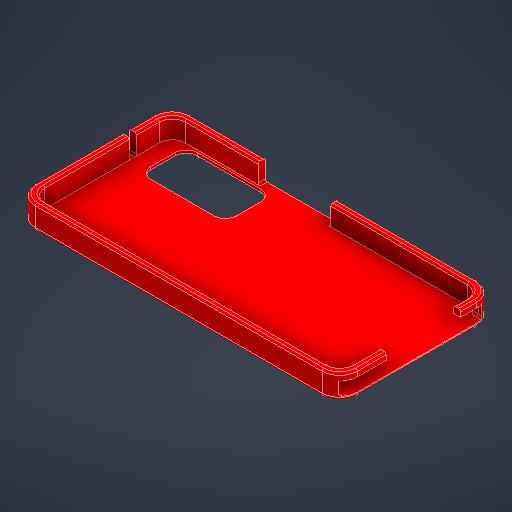
# Autodesk Inventor part: CarcasaBase
Saved by Autodesk Inventor 2026 (Build 300175000, 175)
## iProperties
Created: 2025-06-24
Part Number: CarcasaBase
Material: Genérico
Document SubType Name: Modeling
Designer: Estudiante
Density: 1 g/cm^3
Appearance: Valor por defecto
Author: Estudiante
Autodesk Inventor part; units mm, degrees
ref_plane "YZ Plane" through (0, 0, 0) normal (1, 0, 0) x (0, 1, 0)
ref_plane "XZ Plane" through (0, 0, 0) normal (0, 1, 0) x (-1, 0, 0)
ref_plane "XY Plane" through (0, 0, 0) normal (0, 0, 1) x (1, 0, 0)
sketch "Boceto1" plane through (0, 0, 0) normal (0, 1, 0) x (-1, 0, 0)
  line L0 (0, 0) -> (173, 0)
  line L1 (173, 0) -> (173, -83)
  line L2 (173, -83) -> (0, -83)
  line L3 (0, -83) -> (0, 0)
  dimension "d0" = 173
  dimension "d1" = 83
  constraints: 8 end point, 2 parallel, 1 horizontal, 1 perpendicular
  measures "d0" distance of L1.end L2.end
  measures "d1" distance of L0.end L1.end
extrude "Extrusión1" add sketch "Boceto1" along normal blind 13.2
fillet "Empalme1" radius 9.5 4 edges at (-173, 6.6, -83) (0, 6.6, -83) (-173, 6.6, 0) (0, 6.6, 0)
sketch "Boceto2" plane through (0, 13.2, 0) normal (0, 1, 0) x (1, 0, 0)
  line L0 (0, 0) -> (0, 3.75)
  line L1 (0, 9.5) -> (0, 73.5) projected
  line L2 (0, 3.75) -> (-3.75, 3.75)
  line L3 (-3.75, 3.75) -> (-169.25, 3.75)
  line L4 (-169.25, 3.75) -> (-169.25, 79.25)
  line L5 (-169.25, 79.25) -> (-3.75, 79.25)
  line L6 (-3.75, 79.25) -> (-3.75, 3.75)
  line L7 (-169.25, 3.75) -> (-169.25, 10.75)
  line L8 (-169.25, 10.75) -> (-162.25, 10.75)
  circle A0 centre (-162.25, 10.75) radius 7
  line L9 (-169.25, 79.25) -> (-162.25, 79.25)
  line L10 (-162.25, 79.25) -> (-162.25, 72.25)
  circle A1 centre (-162.25, 72.25) radius 7
  line L11 (-3.75, 3.75) -> (-3.75, 10.75)
  line L12 (-3.75, 10.75) -> (-10.75, 10.75)
  circle A2 centre (-10.75, 10.75) radius 7
  line L13 (-3.75, 79.25) -> (-10.75, 79.25)
  line L14 (-10.75, 79.25) -> (-10.75, 72.25)
  circle A3 centre (-10.75, 72.25) radius 7
  point P0 (-169.25, 72.25)
  point P1 (-162.25, 3.75)
  point P2 (-10.75, 3.75)
  point P3 (-3.75, 72.25)
  dimension "d5" = 3.75
  dimension "d6" = 3.75
  dimension "d7" = 165.5
  dimension "d8" = 75.5
  dimension "d9" = 7
  dimension "d10" = 7
  dimension "d11" = 7
  dimension "d12" = 7
  dimension "d13" = 7
  dimension "d14" = 7
  dimension "d15" = 7
  dimension "d16" = 7
  constraints: 28 end point, 6 perpendicular, 4 coincident, 4 point on line, 2 parallel, 1 collinear, 1 horizontal, 12 other
  measures "d5" distance of L0.start L0.end
  measures "d6" distance of L0.end L2.end
  measures "d7" distance of L4.end L5.end
  measures "d8" distance of L3.end L4.end
  measures "d9" distance of L3.end L7.end
  measures "d10" distance of L7.end L8.end
  measures "d11" distance of L4.end L9.end
  measures "d12" distance of L9.end L10.end
  measures "d13" distance of L2.end L11.end
  measures "d14" distance of L11.end L12.end
  measures "d15" distance of L5.end L13.end
  measures "d16" distance of L13.end L14.end
extrude "Extrusión2" cut sketch "Boceto2" against normal blind 10.7 contours L3 A0 L4 A1 L5 A3 L6 A2 | A2 | A0 | A3 | A1
sketch "Boceto3" plane through (0, 0, 0) normal (0, -1, 0) x (1, 0, 0)
  line L0 (0, 0) -> (0, -65.5)
  line L1 (0, -9.5) -> (0, -73.5) projected
  line L2 (0, -65.5) -> (-137.5, -65.5)
  line L3 (-137.5, -65.5) -> (-137.5, -53)
  line L4 (-137.5, -53) -> (-114.5, -53)
  line L5 (-114.5, -53) -> (-160.5, -53)
  line L6 (-160.5, -53) -> (-160.5, -78)
  line L7 (-160.5, -78) -> (-114.5, -78)
  line L8 (-114.5, -78) -> (-114.5, -53)
  line L9 (-114.5, -78) -> (-114.5, -72)
  line L10 (-114.5, -72) -> (-120.5, -72)
  circle A0 centre (-120.5, -72) radius 6
  line L11 (-114.5, -53) -> (-114.5, -59)
  line L12 (-114.5, -59) -> (-120.5, -59)
  circle A1 centre (-120.5, -59) radius 6
  line L13 (-160.5, -78) -> (-160.5, -72)
  line L14 (-160.5, -72) -> (-154.5, -72)
  circle A2 centre (-154.5, -72) radius 6
  line L15 (-160.5, -53) -> (-154.5, -53)
  line L16 (-154.5, -53) -> (-154.5, -59)
  circle A3 centre (-154.5, -59) radius 6
  point P0 (-160.5, -59)
  point P1 (-154.5, -78)
  point P2 (-120.5, -78)
  point P3 (-120.5, -53)
  dimension "d19" = 65.5
  dimension "d20" = 137.5
  dimension "d21" = 12.5
  dimension "d22" = 23
  dimension "d23" = 46
  dimension "d24" = 25
  dimension "d25" = 6
  dimension "d26" = 6
  dimension "d27" = 6
  dimension "d28" = 6
  dimension "d29" = 6
  dimension "d30" = 6
  dimension "d31" = 6
  dimension "d32" = 6
  constraints: 32 end point, 8 perpendicular, 5 point on line, 4 coincident, 2 parallel, 1 horizontal, 12 other
  measures "d19" distance of L0.start L0.end
  measures "d20" distance of L0.end L2.end
  measures "d21" distance of L2.end L3.end
  measures "d22" distance of L3.end L4.end
  measures "d23" distance of L7.end L6.end
  measures "d24" distance of L6.end L5.end
  measures "d25" distance of L7.end L9.end
  measures "d26" distance of L9.end L10.end
  measures "d27" distance of L4.end L11.end
  measures "d28" distance of L11.end L12.end
  measures "d29" distance of L6.end L13.end
  measures "d30" distance of L13.end L14.end
  measures "d31" distance of L5.end L15.end
  measures "d32" distance of L15.end L16.end
extrude "Extrusión3" cut sketch "Boceto3" against normal blind 2.5 contours L8 A0 L7 A2 L6 A3 L5 L3 L2 | L2 L3 L4 A1 L8 | A0 | A1 | A3 | A2
sketch "Boceto5" plane through (0, 0, -9.5) normal (1, 0, 0) x (0, 0, -1)
  line L0 (-9.5, 0) -> (15.5, 0)
  line L1 (0, 0) -> (64, 0) projected
  line L2 (15.5, 0) -> (15.5, 2.5)
  line L3 (64, 13.2) -> (0, 13.2) projected
  line L4 (15.5, 2.5) -> (55.5, 2.5)
  line L5 (15.5, 2.5) -> (15.5, 13.2)
  line L6 (55.5, 2.5) -> (55.5, 13.2)
  dimension "d38" = 25
  dimension "d39" = 2.5
  dimension "d41" = 40
  constraints: 10 end point, 3 perpendicular, 3 point on line, 1 horizontal
  measures "d38" distance of L0.start L0.end
  measures "d39" distance of L0.end L2.end
  measures "d41" distance of L2.end L4.end
extrude "Extrusión4" cut sketch "Boceto5" against normal blind 13.2
sketch "Boceto6" plane through (-173, 0, -73.5) normal (-1, 0, 0) x (0, 0, 1)
  line L0 (73.5, 0) -> (17.5, 0)
  line L1 (0, 0) -> (64, 0) projected
  line L2 (17.5, 0) -> (17.5, 2.5)
  line L3 (17.5, 2.5) -> (13.5, 2.5)
  line L4 (13.5, 2.5) -> (13.5, 13.2)
  line L5 (0, 13.2) -> (64, 13.2) projected
  line L6 (17.5, 2.5) -> (17.5, 13.2)
  point P0 (29.3, 13.9)
  dimension "d44" = 56
  dimension "d45" = 2.5
  dimension "d46" = 4
  constraints: 10 end point, 3 point on line, 3 vertical, 1 perpendicular
  measures "d44" distance of L0.start L0.end
  measures "d45" distance of L0.end L2.end
  measures "d46" distance of L2.end L3.end
extrude "Extrusión5" cut sketch "Boceto6" against normal blind 10.7
sketch "Boceto7" plane through (-9.5, 0, -83) normal (0, 0, -1) x (-1, 0, 0)
  line L0 (-9.5, 13.2) -> (-9.5, 0) projected
  line L1 (-9.5, 0) -> (74.5, 0)
  line L2 (0, 0) -> (154, 0) projected
  line L3 (74.5, 0) -> (74.5, 2.5)
  line L4 (0, 13.2) -> (154, 13.2) projected
  line L5 (74.5, 2.5) -> (74.5, 13.2)
  line L6 (74.5, 2.5) -> (113.5, 2.5)
  line L7 (1.25, 2.5) -> (152.75, 2.5) projected
  line L8 (113.5, 2.5) -> (113.5, 13.2)
  line L9 (113.5, 13.2) -> (74.5, 13.2)
  dimension "d132" = 84
  dimension "d133" = 2.5
  dimension "d134" = 10.7
  dimension "d135" = 39
  dimension "d136" = 10.7
  constraints: 12 end point, 4 point on line, 1 perpendicular
  measures "d132" distance of L0.end L1.end
  measures "d133" distance of L1.end L3.end
  measures "d134" distance of L3.end L5.end
  measures "d135" distance of L3.end L6.end
  measures "d136" distance of L6.end L8.end
sketch "Boceto12" plane through (0, 2.5, 0) normal (0, 1, 0) x (1, 0, 0)
  line L0 (6.4, 0) -> (6.4, 2.5)
  line L1 (-0.1, 8.5) -> (-0.1, 76.5)
  line L2 (6.4, 2.5) -> (3.9, 2.5)
  line L3 (3.9, 2.5) -> (-164.1, 2.5)
  line L4 (-164.1, 2.5) -> (-164.1, 77.5)
  line L5 (-164.1, 77.5) -> (3.9, 77.5)
  line L6 (3.9, 77.5) -> (3.9, 2.5)
  line L7 (-164.1, 2.5) -> (-164.1, 9.5)
  line L8 (-164.1, 9.5) -> (-157.1, 9.5)
  circle A0 centre (-157.1, 9.5) radius 7
  line L9 (-164.1, 77.5) -> (-157.1, 77.5)
  line L10 (-157.1, 77.5) -> (-157.1, 70.5)
  circle A1 centre (-157.1, 70.5) radius 7
  line L11 (3.9, 2.5) -> (3.9, 9.5)
  line L12 (3.9, 9.5) -> (-3.1, 9.5)
  circle A2 centre (-3.1, 9.5) radius 7
  line L13 (3.9, 77.5) -> (-3.1, 77.5)
  line L14 (-3.1, 77.5) -> (-3.1, 70.5)
  circle A3 centre (-3.1, 70.5) radius 7
  point P0 (0, 0)
  point P1 (-157.1, 2.5)
  point P2 (-3.1, 2.5)
  point P3 (-0.1, 64.1754)
  point P4 (-164.1, 70.5)
  point P5 (-0.1, 15.8246)
  point P6 (-0.1, 76.5)
  point P7 (3.9, 70.5)
  dimension "d90" = 2.5
  dimension "d91" = 2.5
  dimension "d92" = 168
  dimension "d93" = 75
  dimension "d94" = 7
  dimension "d95" = 7
  dimension "d96" = 7
  dimension "d97" = 7
  dimension "d98" = 7
  dimension "d99" = 7
  dimension "d100" = 7
  dimension "d101" = 7
  constraints: 30 end point, 6 perpendicular, 4 coincident, 4 point on line, 3 parallel, 1 horizontal, 12 other
  measures "d90" distance of L0.start L0.end
  measures "d91" distance of L0.end L11.start
  measures "d92" distance of L5.start L6.start
  measures "d93" distance of L3.end L5.start
  measures "d94" distance of L3.end L8.start
  measures "d95" distance of L8.start L8.end
  measures "d96" distance of L5.start L10.start
  measures "d97" distance of L10.start L10.end
  measures "d98" distance of L11.start L11.end
  measures "d99" distance of L11.end L12.end
  measures "d100" distance of L6.start L14.start
  measures "d101" distance of L14.start L14.end
extrude "Extrusión10" cut sketch "Boceto12" along normal blind 7 contours L12 A2 L1 | L1 A2 L12 | A2 L3 A0 L4 A1 L5 A3 L1 | L1 A3 L6 A2 | A3 | A0 | A1
sketch "Boceto9" plane through (-163.5, 0, 0) normal (0, 0, 1) x (1, 0, 0)
  line L0 (154, 0) -> (0, 0) projected
  line L1 (152.75, 2.5) -> (1.25, 2.5) projected
  line L2 (163.5, 0) -> (243.5, 0)
  line L3 (243.5, 0) -> (243.5, 0)
  line L4 (243.5, 0) -> (243.5, 2.5)
  line L5 (243.5, 0) -> (243.5, 2.5)
  line L6 (243.5, 2.5) -> (243.5, 2.5)
  line L7 (243.5, 2.5) -> (243.5, 13.2)
  line L8 (243.5, 13.2) -> (243.5, 13.2)
  line L9 (243.5, 13.2) -> (243.5, 2.5)
  point P0 (243, 2.5)
  point P1 (191, 2.5)
  dimension "d117" = 80
  dimension "d118" = 0
  dimension "d119" = 10.7
  constraints: 16 end point, 6 point on line, 5 perpendicular, 1 collinear
  measures "d117" distance of L2.start L2.end
  measures "d118" distance of L2.end L3.end
  measures "d119" distance of L4.end L7.end
sketch "Boceto10" plane through (0, 0, 0) normal (0, -1, 0) x (1, 0, 0)
  line L0 (0, 0) -> (-102.5, 0)
  line L1 (-163.5, 0) -> (-9.5, 0) projected
  line L2 (-102.5, 0) -> (-102.5, -40)
  line L3 (-102.5, -40) -> (-102.5, -39.99)
  line L4 (-102.5, -39.99) -> (-102.51, -39.99)
  line L5 (-102.51, -39.99) -> (-102.49, -39.99)
  line L6 (-102.49, -39.99) -> (-102.49, -40.01)
  line L7 (-102.49, -40.01) -> (-102.51, -40.01)
  line L8 (-102.51, -40.01) -> (-102.51, -39.99)
  line L9 (-102.51, -40.01) -> (-102.5, -40.01)
  line L10 (-102.5, -40.01) -> (-102.5, -40)
  circle A0 centre (-102.5, -40) radius 0.01
  line L11 (-102.51, -39.99) -> (-102.51, -40)
  line L12 (-102.51, -40) -> (-102.5, -40)
  circle A1 centre (-102.5, -40) radius 0.01
  line L13 (-102.49, -40.01) -> (-102.49, -40)
  line L14 (-102.49, -40) -> (-102.5, -40)
  circle A2 centre (-102.5, -40) radius 0.01
  line L15 (-102.49, -39.99) -> (-102.49, -40)
  line L16 (-102.49, -40) -> (-102.5, -40)
  circle A3 centre (-102.5, -40) radius 0.01
  point P0 (-102.5, -39.99)
  point P1 (-102.5, -39.99)
  point P2 (-102.5, -40.01)
  dimension "d69" = 102.5
  dimension "d70" = 40
  dimension "d71" = 0.01
  dimension "d72" = 0.01
  dimension "d73" = 0.02
  dimension "d74" = 0.02
  dimension "d75" = 0.01
  dimension "d76" = 0.01
  dimension "d77" = 0.01
  dimension "d78" = 0.01
  dimension "d79" = 0.01
  dimension "d80" = 0.01
  dimension "d81" = 0.01
  dimension "d82" = 0.01
  constraints: 32 end point, 6 perpendicular, 4 coincident, 4 midpoint, 2 parallel, 2 point on line, 1 horizontal, 1 vertical, 12 other
  measures "d69" distance of L0.start L0.end
  measures "d70" distance of L0.end L2.end
  measures "d71" distance of L2.end L3.end
  measures "d72" distance of L3.end L4.end
  measures "d73" distance of L6.end L7.end
  measures "d74" distance of L5.end L6.end
  measures "d75" distance of L7.end L9.end
  measures "d76" distance of L9.end L10.end
  measures "d77" distance of L4.end L11.end
  measures "d78" distance of L11.end L12.end
  measures "d79" distance of L6.end L13.end
  measures "d80" distance of L13.end L14.end
  measures "d81" distance of L5.end L15.end
  measures "d82" distance of L15.end L16.end
extrude "Extrusión9" cut sketch "Boceto10" against normal blind 10.7 contours A0 L14 L2 | L2 L12 A0 | L14 A0 L10 | L10 A0 L12
extrude "Extrusión11" [suppressed]
fillet "Empalme15" radius 2 8 edges at (-86.5, 0, 0) (-2.7825, 0, -2.7825) (0, 0, -41.5) (-2.7825, 0, -80.2175) (-86.5, 0, -83) (-170.2175, 0, -80.2175) (-173, 0, -41.5) (-170.2175, 0, -2.7825)
fillet "Empalme16" radius 1 8 edges at (-116.2574, 0, -54.7574) (-114.5, 0, -65.5) (-116.2574, 0, -76.2426) (-137.5, 0, -78) (-158.7426, 0, -76.2426) (-160.5, 0, -65.5) (-158.7426, 0, -54.7574) (-137.5, 0, -53)
fillet "Empalme18" radius 0.01 4 edges at (-102.4929, 0, -40.0071) (-102.5071, 0, -40.0071) (-102.5071, 0, -39.9929) (-102.4929, 0, -39.9929)
fillet "Empalme19" radius 1 10 edges at (-170.2175, 13.2, -2.7825) (-173, 13.2, -32.75) (-86.5, 13.2, 0) (-2.7825, 13.2, -2.7825) (0, 13.2, -17.25) (-2.7825, 13.2, -80.2175) (0, 13.2, -69.25) (-86.5, 13.2, -83) (-170.2175, 13.2, -80.2175) (-173, 13.2, -66.75)
fillet "Empalme20" radius 1 10 edges at (-167.1997, 13.2, -5.8003) (-169.25, 13.2, -33.375) (-86.5, 13.2, -3.75) (-5.8003, 13.2, -5.8003) (-3.75, 13.2, -17.875) (-167.1997, 13.2, -77.1997) (-169.25, 13.2, -66.125) (-86.5, 13.2, -79.25) (-5.8003, 13.2, -77.1997) (-3.75, 13.2, -68.625)
fillet "Empalme21" radius 1 5 edges at (-4.61, 2.5, -77.5) (-1.8805, 2.5, -77.393) (-159.1917, 2.5, -2.8198) (-80.1, 2.5, -2.5) (-3.0887, 2.5, -2.5)
fillet "Empalme22" radius 1 2 edges at (-171.125, 2.5, -56) (-171.125, 2.5, -60)
fillet "Empalme24" [suppressed]
extrude "Extrusión12" cut sketch "Boceto7" against normal blind 5
fillet "Empalme25" radius 1 2 edges at (-123, 2.5, -81.125) (-84, 2.5, -81.125)
equation "\"d9\" = radioEsquina"
equation "\"d10\" = radioEsquina"
equation "\"d11\" = radioEsquina"
equation "\"d12\" = radioEsquina"
equation "\"d13\" = radioEsquina"
equation "\"d14\" = radioEsquina"
equation "\"d15\" = radioEsquina"
equation "\"d16\" = radioEsquina"
equation "\"d25\" = radioCamara"
equation "\"d26\" = radioCamara"
equation "\"d27\" = radioCamara"
equation "\"d28\" = radioCamara"
equation "\"d29\" = radioCamara"
equation "\"d30\" = radioCamara"
equation "\"d31\" = radioCamara"
equation "\"d32\" = radioCamara"
equation "\"d38\" = Xii"
equation "\"d41\" = Xif - Xii"
equation "\"d44\" = Xsi"
equation "\"d46\" = Xsf - Xsi"
equation "\"d93\" = d104"
equation "\"d117\" = Yii"
equation "\"d118\" = Yif - Yii"
equation "\"d71\" = 0.5 * AnchoHuella"
equation "\"d72\" = 0.5 * AltoHuella"
equation "\"d73\" = AltoHuella"
equation "\"d74\" = AnchoHuella"
equation "\"d75\" = RadioHuella"
equation "\"d76\" = RadioHuella"
equation "\"d77\" = RadioHuella"
equation "\"d78\" = RadioHuella"
equation "\"d79\" = RadioHuella"
equation "\"d80\" = RadioHuella"
equation "\"d81\" = RadioHuella"
equation "\"d82\" = RadioHuella"
equation "\"d125\" = RadioEsquinaHuella"
equation "\"Alto\" = 168"
equation "\"Ancho\" = 78"
equation "\"Grosor\" = 8.2"
equation "\"radioEsquina\" = 7"
equation "\"AltoCamara\" = 42"
equation "\"AnchoCamara\" = 21"
equation "\"radioCamara\" = 6"
equation "\"Xcamara\" = 17.5"
equation "\"Ycamara\" = 132.5"
equation "\"Xii\" = 25"
equation "\"Xif\" = 65"
equation "\"Xsf\" = 60"
equation "\"Xsi\" = 56"
equation "\"Yii\" = 80"
equation "\"Yif\" = 80"
equation "\"Ydf\" = 123"
equation "\"Ydi\" = 84"
equation "\"AnchoHuella\" = 0.02"
equation "\"AltoHuella\" = 0.02"
equation "\"RadioHuella\" = 0.01"
equation "\"Xhuella\" = 37.5"
equation "\"RadioEsquinaHuella\" = 0.01"
equation "\"B\" = 0"
equation "\"G\" = 0"
equation "\"pedido\" = 49"
equation "\"d104\" = 75"
